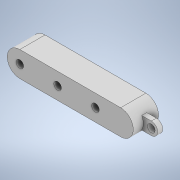
# Autodesk Inventor part: Part7
Saved by Autodesk Inventor 2022 (Build 260153000, 153)
## iProperties
Created: 2022-02-01
Part Number: Part7
Material: Generic
Document SubType Name: Modeling
Designer: br4ch
Density: 1 g/cm^3
Appearance: Default
Author: br4ch
Autodesk Inventor part; units mm, degrees
ref_plane "YZ Plane" through (0, 0, 0) normal (1, 0, 0) x (0, 1, 0)
ref_plane "XZ Plane" through (0, 0, 0) normal (0, 1, 0) x (-1, 0, 0)
sketch "Sketch1" plane through (0, 0, 0) normal (0, 0, 1) x (1, 0, 0)
  line L0 (-13, 4) -> (67, 4) construction
  line L1 (-13, -6) -> (67, -6)
  line L2 (67, 14) -> (-13, 14)
  arc A0 (-13, 14) -> (-13, -6) centre (-13, 4) ccw
  arc A1 (67, -6) -> (67, 14) centre (67, 4) ccw
  circle A2 centre (-13, 4) radius 3
  circle A3 centre (17, 4) radius 3
  circle A4 centre (47, 4) radius 3
  point P0 (0, 0)
  point P1 (27, 4)
  dimension "d0" = 20
  dimension "d16" = 30
  dimension "d17" = 30
  dimension "d18" = 80
  constraints: 7 end point, 5 centre point, 4 point on circle, 4 tangent, 3 point on line, 1 horizontal, 1 midpoint, 1 parallel
  measures "d0" diameter of A1
  measures "d16" distance of L0.start A3.centre
  measures "d17" distance of A4.centre A3.centre
  measures "d18" distance of L0.end A0.centre
extrude "Extrusion1" add sketch "Sketch1" along normal blind 20
ref_plane "Work Plane1" through (0, 0, 10) normal (0, 0, 1) x (1, 0, 0)
sketch "Sketch2" plane through (0, 0, 10) normal (0, 0, 1) x (1, 0, 0)
  arc A0 (67, -6) -> (67, 14) centre (67, 4) ccw projected
  line L0 (67, 14) -> (-13, 14) projected
  arc A1 (-13, 14) -> (-13, -6) centre (-13, 4) ccw projected
  line L1 (-13, -6) -> (67, -6) projected
  arc A2 (67, -6) -> (67, 14) centre (67, 4) ccw projected
  line L2 (65.0126, 4) -> (84.0126, 4) construction
  line L3 (75.6603, 9) -> (83.3215, 9)
  arc A3 (83.3215, -1) -> (83.3215, 9) centre (83.3215, 4) ccw
  line L4 (75.6603, -1) -> (83.3215, -1)
  circle A4 centre (83.3215, 4) radius 3
  point P0 (0, 0)
  point P1 (75.6603, -1)
  dimension "d8" = 10
  dimension "d9" = 6
  constraints: 6 end point, 3 point on circle, 2 centre point, 2 horizontal, 2 point on line, 2 symmetric about line, 1 coincident, 1 tangent
  measures "d8" diameter of A3
  measures "d9" diameter of A4
extrude "Extrusion2" add sketch "Sketch2" along normal mid plane 4 contours A0 L3 A3 L4
equation "\"d6\" = w"
equation "\"d8\" = R"
equation "\"d9\" = r"
equation "\"d10\" = 0.2 * w"
equation "\"r\" = 6"
equation "\"d3\" = 6"
equation "\"d5\" = 6"
equation "\"th\" = 5"
equation "\"R\" = 10"
equation "\"w\" = 20"
body "Solid1"
